Autodesk Inventor part; units mm, degrees
(part 2 of 2)
  spline S229 degree 2 poles (-35.0664, -29.7736) (-35.2121, -29.5414) (-35.3109, -29.0647) (-35.3109, -28.6942) knots 0 0 0 1 2 2 2
  line L272 (-35.3109, -28.6942) -> (-35.3109, -27.9927)
  line L273 (-35.3109, -27.9927) -> (-32.2629, -27.9927)
  line L274 (-32.2629, -27.9927) -> (-32.2629, -28.6868)
  spline S230 degree 2 poles (-32.2629, -28.6868) (-32.2629, -29.1166) (-32.3914, -29.6056) (-32.505, -29.7785) knots 0 0 0 1 2 2 2
  spline S231 degree 2 poles (-32.505, -29.7785) (-32.7001, -30.0725) (-33.3448, -30.396) (-33.7894, -30.396) knots 0 0 0 1 2 2 2
  spline S232 degree 2 poles (-33.7845, -29.9737) (-33.4337, -29.9737) (-32.9372, -29.7415) (-32.7964, -29.5118) knots 0 0 0 1 2 2 2
  spline S233 degree 2 poles (-32.7964, -29.5118) (-32.7001, -29.3488) (-32.6137, -28.9807) (-32.6137, -28.7066) knots 0 0 0 1 2 2 2
  line L275 (-32.6137, -28.7066) -> (-32.6137, -28.3978)
  line L276 (-32.6137, -28.3978) -> (-34.9602, -28.3978)
  line L277 (-34.9602, -28.3978) -> (-34.9602, -28.7066)
  spline S234 degree 2 poles (-34.9602, -28.7066) (-34.9602, -28.9758) (-34.8737, -29.3833) (-34.7576, -29.5488) knots 0 0 0 1 2 2 2
  spline S235 degree 2 poles (-34.7576, -29.5488) (-34.6144, -29.7613) (-34.1401, -29.9737) (-33.7845, -29.9737) knots 0 0 0 1 2 2 2
  spline S236 degree 2 poles (-35.3653, -32.0263) (-35.3653, -31.7299) (-35.1652, -31.2284) (-34.9651, -31.0457) knots 0 0 0 1 2 2 2
  spline S237 degree 2 poles (-34.9651, -31.0457) (-34.7675, -30.8629) (-34.1747, -30.6628) (-33.7894, -30.6628) knots 0 0 0 1 2 2 2
  spline S238 degree 2 poles (-33.7894, -30.6628) (-33.4065, -30.6628) (-32.8384, -30.8579) (-32.6285, -31.0432) knots 0 0 0 1 2 2 2
  spline S239 degree 2 poles (-32.6285, -31.0432) (-32.4235, -31.226) (-32.2086, -31.7249) (-32.2086, -32.0337) knots 0 0 0 1 2 2 2
  spline S240 degree 2 poles (-32.2086, -32.0337) (-32.2086, -32.1868) (-32.253, -32.456) (-32.2876, -32.5697) knots 0 0 0 1 2 2 2
  spline S241 degree 2 poles (-32.2876, -32.5697) (-32.3197, -32.6685) (-32.4111, -32.8735) (-32.4655, -32.9747) knots 0 0 0 1 2 2 2
  line L278 (-32.4655, -32.9747) -> (-32.9545, -32.9747)
  line L279 (-32.9545, -32.9747) -> (-32.9545, -32.9426)
  spline S242 degree 2 poles (-32.9545, -32.9426) (-32.9051, -32.8883) (-32.7668, -32.7203) (-32.7001, -32.5993) knots 0 0 0 1 2 2 2
  spline S243 degree 2 poles (-32.7001, -32.5993) (-32.6359, -32.4832) (-32.5544, -32.209) (-32.5544, -32.0312) knots 0 0 0 1 2 2 2
  spline S244 degree 2 poles (-32.5544, -32.0312) (-32.5544, -31.8361) (-32.7149, -31.4878) (-32.8681, -31.3569) knots 0 0 0 1 2 2 2
  spline S245 degree 2 poles (-32.8681, -31.3569) (-33.0237, -31.2284) (-33.4955, -31.0852) (-33.7894, -31.0852) knots 0 0 0 1 2 2 2
  spline S246 degree 2 poles (-33.7894, -31.0852) (-34.1031, -31.0852) (-34.5551, -31.2359) (-34.7107, -31.3668) knots 0 0 0 1 2 2 2
  spline S247 degree 2 poles (-34.7107, -31.3668) (-34.8614, -31.4952) (-35.0145, -31.8385) (-35.0145, -32.0312) knots 0 0 0 1 2 2 2
  spline S248 degree 2 poles (-35.0145, -32.0312) (-35.0145, -32.2066) (-34.9281, -32.5054) (-34.8638, -32.6215) knots 0 0 0 1 2 2 2
  spline S249 degree 2 poles (-34.8638, -32.6215) (-34.7996, -32.7327) (-34.6662, -32.8982) (-34.6193, -32.9451) knots 0 0 0 1 2 2 2
  line L280 (-34.6193, -32.9451) -> (-34.6193, -32.9747)
  line L281 (-34.6193, -32.9747) -> (-35.1034, -32.9747)
  spline S250 degree 2 poles (-35.1034, -32.9747) (-35.1504, -32.8735) (-35.2368, -32.6956) (-35.2763, -32.5697) knots 0 0 0 1 2 2 2
  spline S251 degree 2 poles (-35.2763, -32.5697) (-35.3208, -32.4363) (-35.3653, -32.209) (-35.3653, -32.0263) knots 0 0 0 1 2 2 2
  spline S252 degree 2 poles (-42.7166, -17.1246) (-42.9142, -17.1246) (-43.2699, -16.9839) (-43.3934, -16.8579) knots 0 0 0 1 2 2 2
  spline S253 degree 2 poles (-43.3934, -16.8579) (-43.549, -16.6998) (-43.7096, -16.2725) (-43.7096, -15.9465) knots 0 0 0 1 2 2 2
  line L282 (-43.7096, -15.9465) -> (-43.7096, -15.6031)
  line L283 (-43.7096, -15.6031) -> (-44.8458, -15.6031)
  line L284 (-44.8458, -15.6031) -> (-44.8458, -15.198)
  line L285 (-44.8458, -15.198) -> (-41.7978, -15.198)
  line L286 (-41.7978, -15.198) -> (-41.7978, -15.9637)
  spline S254 degree 2 poles (-41.7978, -15.9637) (-41.7978, -16.2354) (-41.8867, -16.6158) (-41.988, -16.7616) knots 0 0 0 1 2 2 2
  spline S255 degree 2 poles (-41.988, -16.7616) (-42.1041, -16.932) (-42.4622, -17.1246) (-42.7166, -17.1246) knots 0 0 0 1 2 2 2
  spline S256 degree 2 poles (-42.729, -16.7023) (-42.5709, -16.7023) (-42.3387, -16.5936) (-42.2646, -16.4824) knots 0 0 0 1 2 2 2
  spline S257 degree 2 poles (-42.2646, -16.4824) (-42.2004, -16.3861) (-42.1485, -16.1292) (-42.1485, -15.939) knots 0 0 0 1 2 2 2
  line L287 (-42.1485, -15.939) -> (-42.1485, -15.6031)
  line L288 (-42.1485, -15.6031) -> (-43.3638, -15.6031)
  line L289 (-43.3638, -15.6031) -> (-43.3638, -15.8798)
  spline S258 degree 2 poles (-43.3638, -15.8798) (-43.3638, -16.1268) (-43.2848, -16.4306) (-43.181, -16.5294) knots 0 0 0 1 2 2 2
  spline S259 degree 2 poles (-43.181, -16.5294) (-43.0896, -16.6208) (-42.8747, -16.7023) (-42.729, -16.7023) knots 0 0 0 1 2 2 2
  spline S260 degree 2 poles (-43.7022, -19.36) (-44.2802, -19.36) (-44.91, -18.8043) (-44.91, -18.3399) knots 0 0 0 1 2 2 2
  spline S261 degree 2 poles (-44.91, -18.3399) (-44.91, -17.8632) (-44.2604, -17.3173) (-43.7022, -17.3173) knots 0 0 0 1 2 2 2
  spline S262 degree 2 poles (-43.7022, -17.3173) (-43.1291, -17.3173) (-42.4943, -17.8805) (-42.4943, -18.3399) knots 0 0 0 1 2 2 2
  spline S263 degree 2 poles (-42.4943, -18.3399) (-42.4943, -18.8043) (-43.1267, -19.36) (-43.7022, -19.36) knots 0 0 0 1 2 2 2
  spline S264 degree 2 poles (-43.7022, -18.9623) (-43.2576, -18.9623) (-42.8253, -18.6388) (-42.8253, -18.3399) knots 0 0 0 1 2 2 2
  spline S265 degree 2 poles (-42.8253, -18.3399) (-42.8253, -18.041) (-43.2576, -17.715) (-43.7022, -17.715) knots 0 0 0 1 2 2 2
  spline S266 degree 2 poles (-43.7022, -17.715) (-44.1344, -17.715) (-44.579, -18.041) (-44.579, -18.3399) knots 0 0 0 1 2 2 2
  spline S267 degree 2 poles (-44.579, -18.3399) (-44.579, -18.6363) (-44.1418, -18.9623) (-43.7022, -18.9623) knots 0 0 0 1 2 2 2
  line L290 (-42.5586, -22.5266) -> (-44.8458, -21.9461)
  line L291 (-44.8458, -21.9461) -> (-44.8458, -21.5904)
  line L292 (-44.8458, -21.5904) -> (-43.0822, -21.0322)
  line L293 (-43.0822, -21.0322) -> (-44.8458, -20.4765)
  line L294 (-44.8458, -20.4765) -> (-44.8458, -20.1232)
  line L295 (-44.8458, -20.1232) -> (-42.5586, -19.5379)
  line L296 (-42.5586, -19.5379) -> (-42.5586, -19.938)
  line L297 (-42.5586, -19.938) -> (-44.3296, -20.3431)
  line L298 (-44.3296, -20.3431) -> (-42.5586, -20.884)
  line L299 (-42.5586, -20.884) -> (-42.5586, -21.2026)
  line L300 (-42.5586, -21.2026) -> (-44.3296, -21.7584)
  line L301 (-44.3296, -21.7584) -> (-42.5586, -22.1388)
  line L302 (-42.5586, -22.1388) -> (-42.5586, -22.5266)
  spline S268 degree 2 poles (-44.8977, -23.8579) (-44.8977, -23.3096) (-44.2826, -22.7069) (-43.7145, -22.7069) knots 0 0 0 1 2 2 2
  spline S269 degree 2 poles (-43.7145, -22.7069) (-43.1563, -22.7069) (-42.4943, -23.2923) (-42.4943, -23.7641) knots 0 0 0 1 2 2 2
  spline S270 degree 2 poles (-42.4943, -23.7641) (-42.4943, -23.9765) (-42.6178, -24.305) (-42.7488, -24.426) knots 0 0 0 1 2 2 2
  spline S271 degree 2 poles (-42.7488, -24.426) (-42.8797, -24.5495) (-43.2576, -24.6804) (-43.5318, -24.6804) knots 0 0 0 1 2 2 2
  line L303 (-43.5318, -24.6804) -> (-43.7417, -24.6804)
  line L304 (-43.7417, -24.6804) -> (-43.7417, -23.0971)
  spline S272 degree 2 poles (-43.7417, -23.0971) (-44.1394, -23.0971) (-44.5617, -23.4973) (-44.5617, -23.853) knots 0 0 0 1 2 2 2
  spline S273 degree 2 poles (-44.5617, -23.853) (-44.5617, -23.9789) (-44.5049, -24.2235) (-44.4605, -24.3223) knots 0 0 0 1 2 2 2
  spline S274 degree 2 poles (-44.4605, -24.3223) (-44.4111, -24.426) (-44.3246, -24.5693) (-44.2851, -24.6162) knots 0 0 0 1 2 2 2
  line L305 (-44.2851, -24.6162) -> (-44.2851, -24.6384)
  line L306 (-44.2851, -24.6384) -> (-44.705, -24.6384)
  spline S275 degree 2 poles (-44.705, -24.6384) (-44.7322, -24.5717) (-44.8112, -24.3692) (-44.8335, -24.2902) knots 0 0 0 1 2 2 2
  spline S276 degree 2 poles (-44.8335, -24.2902) (-44.8656, -24.179) (-44.8977, -23.9962) (-44.8977, -23.8579) knots 0 0 0 1 2 2 2
  spline S277 degree 2 poles (-43.4478, -24.305) (-43.2922, -24.3) (-43.0649, -24.2358) (-42.9883, -24.1741) knots 0 0 0 1 2 2 2
  spline S278 degree 2 poles (-42.9883, -24.1741) (-42.9019, -24.1074) (-42.8105, -23.8974) (-42.8105, -23.7418) knots 0 0 0 1 2 2 2
  spline S279 degree 2 poles (-42.8105, -23.7418) (-42.8105, -23.5887) (-42.9019, -23.3738) (-42.9908, -23.2849) knots 0 0 0 1 2 2 2
  spline S280 degree 2 poles (-42.9908, -23.2849) (-43.0822, -23.1984) (-43.302, -23.1095) (-43.4478, -23.0971) knots 0 0 0 1 2 2 2
  line L307 (-43.4478, -23.0971) -> (-43.4478, -24.305)
  line L308 (-42.9711, -26.2835) -> (-42.9711, -26.2637)
  spline S281 degree 2 poles (-42.9711, -26.2637) (-42.9587, -26.2192) (-42.9538, -26.1229) (-42.9538, -26.0562) knots 0 0 0 1 2 2 2
  spline S282 degree 2 poles (-42.9538, -26.0562) (-42.9538, -25.9006) (-43.0896, -25.5943) (-43.223, -25.456) knots 0 0 0 1 2 2 2
  line L309 (-43.223, -25.456) -> (-44.8458, -25.456)
  line L310 (-44.8458, -25.456) -> (-44.8458, -25.0707)
  line L311 (-44.8458, -25.0707) -> (-42.5586, -25.0707)
  line L312 (-42.5586, -25.0707) -> (-42.5586, -25.456)
  line L313 (-42.5586, -25.456) -> (-42.8994, -25.456)
  spline S283 degree 2 poles (-42.8994, -25.456) (-42.7117, -25.666) (-42.5586, -25.9797) (-42.5586, -26.1279) knots 0 0 0 1 2 2 2
  spline S284 degree 2 poles (-42.5586, -26.1279) (-42.5586, -26.1871) (-42.5635, -26.2464) (-42.5709, -26.2835) knots 0 0 0 1 2 2 2
  line L314 (-42.5709, -26.2835) -> (-42.9711, -26.2835)
  spline S285 degree 2 poles (-42.1461, -30.0774) (-42.3486, -30.2503) (-42.9414, -30.443) (-43.3218, -30.443) knots 0 0 0 1 2 2 2
  spline S286 degree 2 poles (-43.3218, -30.443) (-43.6923, -30.443) (-44.2925, -30.2553) (-44.4951, -30.0774) knots 0 0 0 1 2 2 2
  spline S287 degree 2 poles (-44.4951, -30.0774) (-44.7075, -29.8897) (-44.91, -29.3932) (-44.91, -29.0943) knots 0 0 0 1 2 2 2
  spline S288 degree 2 poles (-44.91, -29.0943) (-44.91, -28.7856) (-44.7001, -28.2916) (-44.4951, -28.1113) knots 0 0 0 1 2 2 2
  spline S289 degree 2 poles (-44.4951, -28.1113) (-44.2925, -27.9359) (-43.6972, -27.7482) (-43.3218, -27.7482) knots 0 0 0 1 2 2 2
  spline S290 degree 2 poles (-43.3218, -27.7482) (-42.9389, -27.7482) (-42.356, -27.9384) (-42.1461, -28.1138) knots 0 0 0 1 2 2 2
  spline S291 degree 2 poles (-42.1461, -28.1138) (-41.9435, -28.2916) (-41.7336, -28.7881) (-41.7336, -29.0943) knots 0 0 0 1 2 2 2
  spline S292 degree 2 poles (-41.7336, -29.0943) (-41.7336, -29.4056) (-41.9509, -29.9045) (-42.1461, -30.0774) knots 0 0 0 1 2 2 2
  spline S293 degree 2 poles (-43.3218, -30.0206) (-43.0205, -30.0206) (-42.5536, -29.8897) (-42.4005, -29.7711) knots 0 0 0 1 2 2 2
  spline S294 degree 2 poles (-42.4005, -29.7711) (-42.2424, -29.6501) (-42.0843, -29.3092) (-42.0843, -29.0968) knots 0 0 0 1 2 2 2
  spline S295 degree 2 poles (-42.0843, -29.0968) (-42.0843, -28.877) (-42.2375, -28.546) (-42.4005, -28.42) knots 0 0 0 1 2 2 2
  spline S296 degree 2 poles (-42.4005, -28.42) (-42.5561, -28.299) (-43.0254, -28.1706) (-43.3218, -28.1706) knots 0 0 0 1 2 2 2
  spline S297 degree 2 poles (-43.3218, -28.1706) (-43.922, -28.1706) (-44.5593, -28.6744) (-44.5593, -29.0968) knots 0 0 0 1 2 2 2
  spline S298 degree 2 poles (-44.5593, -29.0968) (-44.5593, -29.5192) (-43.922, -30.0206) (-43.3218, -30.0206) knots 0 0 0 1 2 2 2
  line L315 (-44.8458, -33.1106) -> (-44.8458, -32.5845)
  line L316 (-44.8458, -32.5845) -> (-43.428, -31.4705)
  line L317 (-43.428, -31.4705) -> (-43.6281, -31.2927)
  line L318 (-43.6281, -31.2927) -> (-44.8458, -31.2927)
  line L319 (-44.8458, -31.2927) -> (-44.8458, -30.8876)
  line L320 (-44.8458, -30.8876) -> (-41.7978, -30.8876)
  line L321 (-41.7978, -30.8876) -> (-41.7978, -31.2927)
  line L322 (-41.7978, -31.2927) -> (-43.1983, -31.2927)
  line L323 (-43.1983, -31.2927) -> (-41.7978, -32.5425)
  line L324 (-41.7978, -32.5425) -> (-41.7978, -33.0365)
  line L325 (-41.7978, -33.0365) -> (-43.1588, -31.7743)
  line L326 (-43.1588, -31.7743) -> (-44.8458, -33.1106)
  line L327 (-53.1901, -24.3223) -> (-53.1901, -23.2898)
  line L328 (-53.1901, -23.2898) -> (-54.2226, -23.2898)
  line L329 (-54.2226, -23.2898) -> (-54.2226, -22.9489)
  line L330 (-54.2226, -22.9489) -> (-53.1901, -22.9489)
  line L331 (-53.1901, -22.9489) -> (-53.1901, -21.9165)
  line L332 (-53.1901, -21.9165) -> (-52.8616, -21.9165)
  line L333 (-52.8616, -21.9165) -> (-52.8616, -22.9489)
  line L334 (-52.8616, -22.9489) -> (-51.8292, -22.9489)
  line L335 (-51.8292, -22.9489) -> (-51.8292, -23.2898)
  line L336 (-51.8292, -23.2898) -> (-52.8616, -23.2898)
  line L337 (-52.8616, -23.2898) -> (-52.8616, -24.3223)
  line L338 (-52.8616, -24.3223) -> (-53.1901, -24.3223)
  spline S299 degree 2 poles (-53.3927, -26.7133) (-53.6125, -26.7133) (-53.9879, -26.5725) (-54.1263, -26.444) knots 0 0 0 1 2 2 2
  spline S300 degree 2 poles (-54.1263, -26.444) (-54.2646, -26.3156) (-54.4251, -25.9327) (-54.4251, -25.6956) knots 0 0 0 1 2 2 2
  spline S301 degree 2 poles (-54.4251, -25.6956) (-54.4251, -25.4782) (-54.3288, -25.0534) (-54.2522, -24.8978) knots 0 0 0 1 2 2 2
  line L339 (-54.2522, -24.8978) -> (-53.82, -24.8978)
  line L340 (-53.82, -24.8978) -> (-53.82, -24.9274)
  spline S302 degree 2 poles (-53.82, -24.9274) (-53.8546, -24.9744) (-53.9435, -25.1497) (-53.983, -25.2559) knots 0 0 0 1 2 2 2
  spline S303 degree 2 poles (-53.983, -25.2559) (-54.025, -25.377) (-54.0719, -25.577) (-54.0719, -25.703) knots 0 0 0 1 2 2 2
  spline S304 degree 2 poles (-54.0719, -25.703) (-54.0719, -25.8265) (-53.983, -26.0587) (-53.8867, -26.1427) knots 0 0 0 1 2 2 2
  spline S305 degree 2 poles (-53.8867, -26.1427) (-53.7953, -26.2192) (-53.5532, -26.2983) (-53.3902, -26.2983) knots 0 0 0 1 2 2 2
  spline S306 degree 2 poles (-53.3902, -26.2983) (-53.2272, -26.2983) (-53.0197, -26.2094) (-52.9505, -26.1254) knots 0 0 0 1 2 2 2
  spline S307 degree 2 poles (-52.9505, -26.1254) (-52.874, -26.0389) (-52.8098, -25.7821) (-52.8098, -25.6264) knots 0 0 0 1 2 2 2
  spline S308 degree 2 poles (-52.8098, -25.6264) (-52.8098, -25.4585) (-52.8616, -25.125) (-52.8839, -25.0238) knots 0 0 0 1 2 2 2
  line L341 (-52.8839, -25.0238) -> (-51.3129, -25.0238)
  line L342 (-51.3129, -25.0238) -> (-51.3129, -26.696)
  line L343 (-51.3129, -26.696) -> (-51.6711, -26.696)
  line L344 (-51.6711, -26.696) -> (-51.6711, -25.4165)
  line L345 (-51.6711, -25.4165) -> (-52.4837, -25.4165)
  spline S309 degree 2 poles (-52.4837, -25.4165) (-52.4738, -25.4906) (-52.4664, -25.6339) (-52.4664, -25.6931) knots 0 0 0 1 2 2 2
  spline S310 degree 2 poles (-52.4664, -25.6931) (-52.4664, -25.9278) (-52.543, -26.2514) (-52.6566, -26.3996) knots 0 0 0 1 2 2 2
  spline S311 degree 2 poles (-52.6566, -26.3996) (-52.7702, -26.5502) (-53.116, -26.7133) (-53.3927, -26.7133) knots 0 0 0 1 2 2 2
  spline S312 degree 2 poles (-54.4153, -29.3982) (-54.4153, -29.0672) (-54.2769, -28.6028) (-54.1781, -28.3978) knots 0 0 0 1 2 2 2
  line L346 (-54.1781, -28.3978) -> (-53.6693, -28.3978)
  line L347 (-53.6693, -28.3978) -> (-53.6693, -28.4274)
  spline S313 degree 2 poles (-53.6693, -28.4274) (-53.857, -28.6275) (-54.0645, -29.1339) (-54.0645, -29.3685) knots 0 0 0 1 2 2 2
  spline S314 degree 2 poles (-54.0645, -29.3685) (-54.0645, -29.7044) (-53.7854, -30.0478) (-53.5557, -30.0478) knots 0 0 0 1 2 2 2
  spline S315 degree 2 poles (-53.5557, -30.0478) (-53.3729, -30.0478) (-53.1457, -29.8675) (-53.0889, -29.6723) knots 0 0 0 1 2 2 2
  spline S316 degree 2 poles (-53.0889, -29.6723) (-53.0493, -29.5315) (-52.995, -29.2969) (-52.9505, -29.1215) knots 0 0 0 1 2 2 2
  spline S317 degree 2 poles (-52.9505, -29.1215) (-52.9086, -28.9634) (-52.7826, -28.714) (-52.6813, -28.6176) knots 0 0 0 1 2 2 2
  spline S318 degree 2 poles (-52.6813, -28.6176) (-52.58, -28.5238) (-52.3083, -28.42) (-52.1305, -28.42) knots 0 0 0 1 2 2 2
  spline S319 degree 2 poles (-52.1305, -28.42) (-51.76, -28.42) (-51.2586, -28.998) (-51.2586, -29.4451) knots 0 0 0 1 2 2 2
  spline S320 degree 2 poles (-51.2586, -29.4451) (-51.2586, -29.702) (-51.3599, -30.1565) (-51.4562, -30.3516) knots 0 0 0 1 2 2 2
  line L348 (-51.4562, -30.3516) -> (-51.9403, -30.3516)
  line L349 (-51.9403, -30.3516) -> (-51.9403, -30.3219)
  spline S321 degree 2 poles (-51.9403, -30.3219) (-51.8069, -30.1762) (-51.6093, -29.7217) (-51.6093, -29.4723) knots 0 0 0 1 2 2 2
  spline S322 degree 2 poles (-51.6093, -29.4723) (-51.6093, -29.1907) (-51.8736, -28.8424) (-52.0885, -28.8424) knots 0 0 0 1 2 2 2
  spline S323 degree 2 poles (-52.0885, -28.8424) (-52.2812, -28.8424) (-52.5109, -29.0474) (-52.5627, -29.2401) knots 0 0 0 1 2 2 2
  spline S324 degree 2 poles (-52.5627, -29.2401) (-52.5973, -29.3685) (-52.6863, -29.7415) (-52.7233, -29.865) knots 0 0 0 1 2 2 2
  spline S325 degree 2 poles (-52.7233, -29.865) (-52.8196, -30.1787) (-53.2074, -30.4701) (-53.4915, -30.4701) knots 0 0 0 1 2 2 2
  spline S326 degree 2 poles (-53.4915, -30.4701) (-53.6718, -30.4701) (-54.0176, -30.3244) (-54.1386, -30.1935) knots 0 0 0 1 2 2 2
  spline S327 degree 2 poles (-54.1386, -30.1935) (-54.272, -30.0478) (-54.4153, -29.6773) (-54.4153, -29.3982) knots 0 0 0 1 2 2 2
  spline S328 degree 2 poles (-53.4248, -32.95) (-53.652, -32.95) (-54.0003, -32.7771) (-54.1139, -32.6339) knots 0 0 0 1 2 2 2
  spline S329 degree 2 poles (-54.1139, -32.6339) (-54.2473, -32.461) (-54.3609, -32.0682) (-54.3609, -31.757) knots 0 0 0 1 2 2 2
  line L350 (-54.3609, -31.757) -> (-54.3609, -30.8826)
  line L351 (-54.3609, -30.8826) -> (-51.3129, -30.8826)
  line L352 (-51.3129, -30.8826) -> (-51.3129, -31.6903)
  spline S330 degree 2 poles (-51.3129, -31.6903) (-51.3129, -32.0164) (-51.3549, -32.3424) (-51.4364, -32.4906) knots 0 0 0 1 2 2 2
  spline S331 degree 2 poles (-51.4364, -32.4906) (-51.5229, -32.6561) (-51.8069, -32.8068) (-51.9996, -32.8068) knots 0 0 0 1 2 2 2
  spline S332 degree 2 poles (-51.9996, -32.8068) (-52.2145, -32.8068) (-52.5553, -32.5795) (-52.6517, -32.3795) knots 0 0 0 1 2 2 2
  line L353 (-52.6517, -32.3795) -> (-52.6665, -32.3795)
  spline S333 degree 2 poles (-52.6665, -32.3795) (-52.7406, -32.6512) (-53.1333, -32.95) (-53.4248, -32.95) knots 0 0 0 1 2 2 2
  spline S334 degree 2 poles (-53.4421, -32.5277) (-53.2692, -32.5277) (-53.0469, -32.4289) (-52.9678, -32.2807) knots 0 0 0 1 2 2 2
  spline S335 degree 2 poles (-52.9678, -32.2807) (-52.9184, -32.1843) (-52.8888, -31.9571) (-52.8888, -31.7471) knots 0 0 0 1 2 2 2
  line L354 (-52.8888, -31.7471) -> (-52.8888, -31.2877)
  line L355 (-52.8888, -31.2877) -> (-54.0151, -31.2877)
  line L356 (-54.0151, -31.2877) -> (-54.0151, -31.6162)
  spline S336 degree 2 poles (-54.0151, -31.6162) (-54.0151, -31.883) (-53.9657, -32.1893) (-53.8867, -32.3078) knots 0 0 0 1 2 2 2
  spline S337 degree 2 poles (-53.8867, -32.3078) (-53.8052, -32.4215) (-53.6026, -32.5277) (-53.4421, -32.5277) knots 0 0 0 1 2 2 2
  spline S338 degree 2 poles (-52.0564, -32.3844) (-51.9477, -32.3844) (-51.7847, -32.3103) (-51.7378, -32.2288) knots 0 0 0 1 2 2 2
  spline S339 degree 2 poles (-51.7378, -32.2288) (-51.6834, -32.13) (-51.6587, -31.8904) (-51.6587, -31.6755) knots 0 0 0 1 2 2 2
  line L357 (-51.6587, -31.6755) -> (-51.6587, -31.2877)
  line L358 (-51.6587, -31.2877) -> (-52.5504, -31.2877)
  line L359 (-52.5504, -31.2877) -> (-52.5504, -31.7471)
  spline S340 degree 2 poles (-52.5504, -31.7471) (-52.5504, -31.9373) (-52.5109, -32.1176) (-52.4491, -32.214) knots 0 0 0 1 2 2 2
  spline S341 degree 2 poles (-52.4491, -32.214) (-52.3898, -32.3078) (-52.1997, -32.3844) (-52.0564, -32.3844) knots 0 0 0 1 2 2 2
  spline S342 degree 2 poles (-61.7666, -23.559) (-61.9642, -23.559) (-62.3199, -23.4183) (-62.4434, -23.2923) knots 0 0 0 1 2 2 2
  spline S343 degree 2 poles (-62.4434, -23.2923) (-62.599, -23.1342) (-62.7596, -22.7069) (-62.7596, -22.3808) knots 0 0 0 1 2 2 2
  line L360 (-62.7596, -22.3808) -> (-62.7596, -22.0375)
  line L361 (-62.7596, -22.0375) -> (-63.8958, -22.0375)
  line L362 (-63.8958, -22.0375) -> (-63.8958, -21.6324)
  line L363 (-63.8958, -21.6324) -> (-60.8478, -21.6324)
  line L364 (-60.8478, -21.6324) -> (-60.8478, -22.3981)
  spline S344 degree 2 poles (-60.8478, -22.3981) (-60.8478, -22.6698) (-60.9367, -23.0502) (-61.038, -23.1959) knots 0 0 0 1 2 2 2
  spline S345 degree 2 poles (-61.038, -23.1959) (-61.1541, -23.3664) (-61.5122, -23.559) (-61.7666, -23.559) knots 0 0 0 1 2 2 2
  spline S346 degree 2 poles (-61.779, -23.1367) (-61.6209, -23.1367) (-61.3887, -23.028) (-61.3146, -22.9168) knots 0 0 0 1 2 2 2
  spline S347 degree 2 poles (-61.3146, -22.9168) (-61.2504, -22.8205) (-61.1985, -22.5636) (-61.1985, -22.3734) knots 0 0 0 1 2 2 2
  line L365 (-61.1985, -22.3734) -> (-61.1985, -22.0375)
  line L366 (-61.1985, -22.0375) -> (-62.4138, -22.0375)
  line L367 (-62.4138, -22.0375) -> (-62.4138, -22.3142)
  spline S348 degree 2 poles (-62.4138, -22.3142) (-62.4138, -22.5612) (-62.3348, -22.865) (-62.231, -22.9638) knots 0 0 0 1 2 2 2
  spline S349 degree 2 poles (-62.231, -22.9638) (-62.1396, -23.0552) (-61.9247, -23.1367) (-61.779, -23.1367) knots 0 0 0 1 2 2 2
  spline S350 degree 2 poles (-63.9501, -24.794) (-63.9501, -24.4631) (-63.8118, -23.9987) (-63.713, -23.7937) knots 0 0 0 1 2 2 2
  line L368 (-63.713, -23.7937) -> (-63.2042, -23.7937)
  line L369 (-63.2042, -23.7937) -> (-63.2042, -23.8233)
  spline S351 degree 2 poles (-63.2042, -23.8233) (-63.3919, -24.0234) (-63.5994, -24.5298) (-63.5994, -24.7644) knots 0 0 0 1 2 2 2
  spline S352 degree 2 poles (-63.5994, -24.7644) (-63.5994, -25.1003) (-63.3203, -25.4437) (-63.0906, -25.4437) knots 0 0 0 1 2 2 2
  spline S353 degree 2 poles (-63.0906, -25.4437) (-62.9078, -25.4437) (-62.6806, -25.2634) (-62.6237, -25.0682) knots 0 0 0 1 2 2 2
  spline S354 degree 2 poles (-62.6237, -25.0682) (-62.5842, -24.9274) (-62.5299, -24.6928) (-62.4854, -24.5174) knots 0 0 0 1 2 2 2
  spline S355 degree 2 poles (-62.4854, -24.5174) (-62.4434, -24.3593) (-62.3175, -24.1099) (-62.2162, -24.0135) knots 0 0 0 1 2 2 2
  spline S356 degree 2 poles (-62.2162, -24.0135) (-62.1149, -23.9197) (-61.8432, -23.8159) (-61.6654, -23.8159) knots 0 0 0 1 2 2 2
  spline S357 degree 2 poles (-61.6654, -23.8159) (-61.2949, -23.8159) (-60.7935, -24.3939) (-60.7935, -24.841) knots 0 0 0 1 2 2 2
  spline S358 degree 2 poles (-60.7935, -24.841) (-60.7935, -25.0979) (-60.8947, -25.5523) (-60.9911, -25.7475) knots 0 0 0 1 2 2 2
  line L370 (-60.9911, -25.7475) -> (-61.4752, -25.7475)
  line L371 (-61.4752, -25.7475) -> (-61.4752, -25.7178)
  spline S359 degree 2 poles (-61.4752, -25.7178) (-61.3418, -25.5721) (-61.1442, -25.1176) (-61.1442, -24.8681) knots 0 0 0 1 2 2 2
  spline S360 degree 2 poles (-61.1442, -24.8681) (-61.1442, -24.5866) (-61.4085, -24.2383) (-61.6234, -24.2383) knots 0 0 0 1 2 2 2
  spline S361 degree 2 poles (-61.6234, -24.2383) (-61.816, -24.2383) (-62.0458, -24.4433) (-62.0976, -24.636) knots 0 0 0 1 2 2 2
  spline S362 degree 2 poles (-62.0976, -24.636) (-62.1322, -24.7644) (-62.2211, -25.1374) (-62.2582, -25.2609) knots 0 0 0 1 2 2 2
  spline S363 degree 2 poles (-62.2582, -25.2609) (-62.3545, -25.5746) (-62.7423, -25.866) (-63.0264, -25.866) knots 0 0 0 1 2 2 2
  spline S364 degree 2 poles (-63.0264, -25.866) (-63.2067, -25.866) (-63.5525, -25.7203) (-63.6735, -25.5894) knots 0 0 0 1 2 2 2
  spline S365 degree 2 poles (-63.6735, -25.5894) (-63.8069, -25.4437) (-63.9501, -25.0732) (-63.9501, -24.794) knots 0 0 0 1 2 2 2
  spline S366 degree 2 poles (-61.1961, -29.744) (-61.3986, -29.9169) (-61.9914, -30.1095) (-62.3718, -30.1095) knots 0 0 0 1 2 2 2
  spline S367 degree 2 poles (-62.3718, -30.1095) (-62.7423, -30.1095) (-63.3425, -29.9218) (-63.5451, -29.744) knots 0 0 0 1 2 2 2
  spline S368 degree 2 poles (-63.5451, -29.744) (-63.7575, -29.5562) (-63.96, -29.0598) (-63.96, -28.7609) knots 0 0 0 1 2 2 2
  spline S369 degree 2 poles (-63.96, -28.7609) (-63.96, -28.4521) (-63.7501, -27.9581) (-63.5451, -27.7778) knots 0 0 0 1 2 2 2
  spline S370 degree 2 poles (-63.5451, -27.7778) (-63.3425, -27.6025) (-62.7472, -27.4147) (-62.3718, -27.4147) knots 0 0 0 1 2 2 2
  spline S371 degree 2 poles (-62.3718, -27.4147) (-61.9889, -27.4147) (-61.406, -27.6049) (-61.1961, -27.7803) knots 0 0 0 1 2 2 2
  spline S372 degree 2 poles (-61.1961, -27.7803) (-60.9935, -27.9581) (-60.7836, -28.4546) (-60.7836, -28.7609) knots 0 0 0 1 2 2 2
  spline S373 degree 2 poles (-60.7836, -28.7609) (-60.7836, -29.0721) (-61.0009, -29.5711) (-61.1961, -29.744) knots 0 0 0 1 2 2 2
  spline S374 degree 2 poles (-62.3718, -29.6872) (-62.0705, -29.6872) (-61.6036, -29.5562) (-61.4505, -29.4377) knots 0 0 0 1 2 2 2
  spline S375 degree 2 poles (-61.4505, -29.4377) (-61.2924, -29.3166) (-61.1343, -28.9758) (-61.1343, -28.7634) knots 0 0 0 1 2 2 2
  spline S376 degree 2 poles (-61.1343, -28.7634) (-61.1343, -28.5435) (-61.2875, -28.2126) (-61.4505, -28.0866) knots 0 0 0 1 2 2 2
  spline S377 degree 2 poles (-61.4505, -28.0866) (-61.6061, -27.9655) (-62.0754, -27.8371) (-62.3718, -27.8371) knots 0 0 0 1 2 2 2
  spline S378 degree 2 poles (-62.3718, -27.8371) (-62.972, -27.8371) (-63.6093, -28.341) (-63.6093, -28.7634) knots 0 0 0 1 2 2 2
  spline S379 degree 2 poles (-63.6093, -28.7634) (-63.6093, -29.1857) (-62.972, -29.6872) (-62.3718, -29.6872) knots 0 0 0 1 2 2 2
  line L372 (-63.8958, -32.7352) -> (-63.8958, -32.2807)
  line L373 (-63.8958, -32.2807) -> (-61.2677, -30.932)
  line L374 (-61.2677, -30.932) -> (-63.8958, -30.932)
  line L375 (-63.8958, -30.932) -> (-63.8958, -30.5541)
  line L376 (-63.8958, -30.5541) -> (-60.8478, -30.5541)
  line L377 (-60.8478, -30.5541) -> (-60.8478, -31.1296)
  line L378 (-60.8478, -31.1296) -> (-63.261, -32.3572)
  line L379 (-63.261, -32.3572) -> (-60.8478, -32.3572)
  line L380 (-60.8478, -32.3572) -> (-60.8478, -32.7352)
  line L381 (-60.8478, -32.7352) -> (-63.8958, -32.7352)
  point P0 (58.2782, -33.0439)
  point P1 (42.4032, -33.0439)
  point P2 (26.5282, -33.0439)
  point P3 (10.6532, -33.0439)
  point P4 (-5.2218, -33.0439)
  point P5 (-21.0968, -33.0439)
  point P6 (-33.7968, -33.0439)
  point P7 (-43.3218, -33.0439)
  point P8 (-52.8468, -33.0439)
  point P9 (-62.3718, -33.0439)
  dimension "d22" = 0
  dimension "d42" = 3.1764
  constraints: 10 midpoint, 10 vertical alignment, 9 horizontal alignment, 1 parallel, 20 other
  measures "d42" distance of L1.end L2.end
emboss "Emboss1" sketch "Sketch2" operation add depth 0.254 direction (0, 0, -1) contours L41 L42 L43 L44 L45 L46 L47 L48 L49 L50 L51 L52 | S0 S1 L53 L54 S2 S3 S4 S5 L55 S6 S7 S8 S9 S10 L56 L57 S11 S12 S13 S14 S15 L58 L59 L60 S16 S17 S18 | L61 L62 L63 L64 | S19 S20 L65 L66 S21 S22 S23 S24 L67 S25 S26 S27 S28 S29 L68 L69 S30 S31 S32 S33 S34 L70 L71 L72 S35 S36 S37 | L73 L74 L75 L76 L77 L78 L79 | S38 S39 L80 L81 L82 S40 S41 | S46 S47 S48 S49 S50 S51 L86 L87 S52 S53 S54 S55 S56 S57 S58 S59 L88 L89 S60 S61 | L90 L91 L92 L93 L94 L95 L96 L97 L98 L99 L100 L101 | S62 S63 S64 L102 L103 S65 S66 S67 S68 S69 S70 S71 L104 L105 L106 L107 L108 S72 S73 S74 | L109 L110 L111 L112 L113 L114 L115 | S75 S76 L116 L117 L118 S77 S78 | S83 S84 S85 S86 S87 S88 L122 L123 S89 S90 S91 S92 S93 S94 S95 S96 L124 L125 S97 S98 | S99 S100 S101 S102 S103 S104 L126 L127 S105 S106 S107 S108 S109 S110 L128 L129 L130 L131 L132 S111 S112 | L133 L134 L135 L136 L137 L138 L139 L140 L141 L142 | S113 S114 L143 L144 L145 S115 S116 | S121 S122 S123 S124 S125 S126 L149 L150 S127 S128 S129 S130 S131 S132 L151 L152 L153 L154 L155 S133 S134 | L156 L157 L158 L159 L160 L161 L162 L163 L164 L165 | S135 S136 L166 L167 L168 S137 S138 | L172 L173 L174 L175 L176 L177 L178 L179 L180 L181 L182 L183 | L184 L185 L186 L187 L188 L189 S143 L190 L191 L192 L193 | L194 L195 S144 S145 S146 S147 S148 S149 L196 L197 S150 S151 S152 S153 S154 L198 L199 | L200 L201 L202 L203 L204 L205 L206 | S155 S156 L207 L208 L209 S157 S158 | S163 S164 S165 S166 S167 S168 L213 L214 S169 S170 S171 S172 S173 S174 S175 S176 L215 L216 S177 S178 | L217 L218 L219 L220 | L221 L222 L223 L224 L225 L226 S179 L227 L228 L229 L230 | L231 L232 S180 S181 S182 S183 S184 S185 L233 L234 S186 S187 S188 S189 S190 L235 L236 | L237 L238 L239 L240 L241 L242 L243 | S191 S192 L244 L245 L246 S193 S194 | S199 S200 S201 S202 S203 S204 L250 L251 S205 S206 S207 S208 S209 S210 S211 S212 L252 L253 S213 S214 | L254 L255 L256 L257 | S215 S216 S217 L258 L259 S218 S219 S220 S221 S222 S223 S224 L260 L261 L262 L263 L264 S225 S226 S227 | L265 L266 L267 L268 L269 L270 L271 | S228 S229 L272 L273 L274 S230 S231 | S236 S237 S238 S239 S240 S241 L278 L279 S242 S243 S244 S245 S246 S247 S248 S249 L280 L281 S250 S251 | S252 S253 L282 L283 L284 L285 L286 S254 S255 | S260 S261 S262 S263 | L290 L291 L292 L293 L294 L295 L296 L297 L298 L299 L300 L301 L302 | S268 S269 S270 S271 L303 L304 S272 S273 S274 L305 L306 S275 S276 | L308 S281 S282 L309 L310 L311 L312 L313 S283 S284 L314 | S285 S286 S287 S288 S289 S290 S291 S292 | L315 L316 L317 L318 L319 L320 L321 L322 L323 L324 L325 L326 | L327 L328 L329 L330 L331 L332 L333 L334 L335 L336 L337 L338 | S299 S300 S301 L339 L340 S302 S303 S304 S305 S306 S307 S308 L341 L342 L343 L344 L345 S309 S310 S311 | S312 L346 L347 S313 S314 S315 S316 S317 S318 S319 S320 L348 L349 S321 S322 S323 S324 S325 S326 S327 | S328 S329 L350 L351 L352 S330 S331 S332 L353 S333 | S342 S343 L360 L361 L362 L363 L364 S344 S345 | S350 L368 L369 S351 S352 S353 S354 S355 S356 S357 S358 L370 L371 S359 S360 S361 S362 S363 S364 S365 | S366 S367 S368 S369 S370 S371 S372 S373 | L372 L373 L374 L375 L376 L377 L378 L379 L380 L381
body "Solid1"
